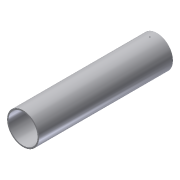
# Autodesk Inventor part: sleeve_spar_ONLY
Saved by Autodesk Inventor 2015 (Build 190159000, 159)
## iProperties
Company: HERA Project
Created: 2013-05-14
Part Number: sleeve_spar_ONLY
Material: PVC-Piping
Document SubType Name: Modeling
Designer: David DeBoer
Density: 1.4 g/cm^3
Mass: 429.807 g
Surface Area: 1214.86 cm^2
Volume: 307.005 cm^3
Description: Hub mating sleeve
Appearance: Smooth - White
Author: David DeBoer
Title: Hub mating sleeve
Autodesk Inventor part; units mm, degrees
ref_plane "YZ Plane" through (0, 0, 0) normal (1, 0, 0) x (0, 1, 0)
ref_plane "XZ Plane" through (0, 0, 0) normal (0, 1, 0) x (-1, 0, 0)
sketch "Sketch1" plane through (0, 0, 0) normal (0, 0, 1) x (1, 0, 0)
  circle A0 centre (0, 0) radius 45
  circle A1 centre (0, 0) radius 41.1
  dimension "d0" = 90
  dimension "d2" = 3.9
  constraints: 2 centre point, 1 coincident
  measures "d0" diameter of A0
  measures "d2" radial gap between concentric circles of A1 A0
extrude "Extrusion1" add sketch "Sketch1" along normal blind 377
sketch "Sketch2" plane through (0, 0, 377) normal (0, 0, 1) x (1, 0, 0)
  circle A0 centre (0, 0) radius 41.1 projected
  circle A1 centre (0, 0) radius 45 projected
  point P0 (0, 45)
  constraints: 1 vertical alignment, 1 other
ref_plane "Work Plane1" through (0, 45, 377) normal (0, 1, 0) x (-1, 0, 0)
sketch "Sketch5" plane through (0, 45, 377) normal (0, 1, 0) x (-1, 0, 0)
  circle A0 centre (0, -357) radius 4.4901
  point P0 (0, -377)
  dimension "d25" = 20
  constraints: 1 centre point
  measures "d25" distance of point (0, -377) A0.centre
hole "nailHole" at (0, 45, 20) direction (0, -1, 0) diameter 3.175 end through all
equation "\"d0\" = sleeveOD"
equation "\"d2\" = sleeveWall"
equation "\"d3\" = sleeveLength"
equation "\"d25\" = nailDelta"
equation "\"sleeveOD\" = 90"
equation "\"sleeveWall\" = 3.9"
equation "\"sleeveLength\" = 377"
equation "\"nailDelta\" = 20"
equation "\"sparLaunchAngle\" = 3.72deg"
body "Solid1"
